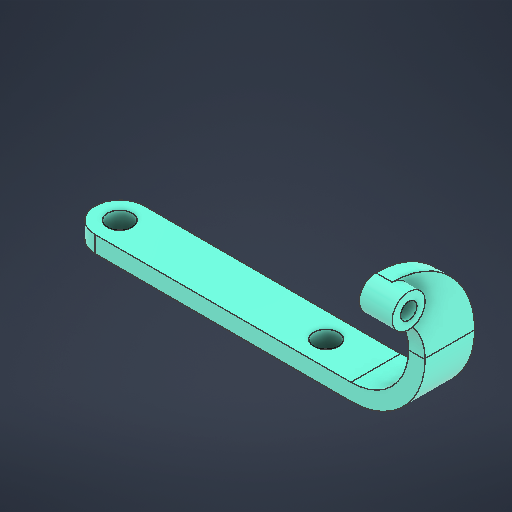
# Autodesk Inventor part: electronics_holder2
Saved by Autodesk Inventor 2026.1 (Build 301233000, 233)
## iProperties
Created: 2025-12-23
Part Number: electronics_holder2
Material: Generic
Document SubType Name: Modeling
Designer: emanuel
Density: 1 g/cm^3
Appearance: Default
Author: emanuel
Autodesk Inventor part; units mm, degrees
ref_plane "YZ Plane" through (0, 0, 0) normal (1, 0, 0) x (0, 1, 0)
ref_plane "XZ Plane" through (0, 0, 0) normal (0, 1, 0) x (-1, 0, 0)
ref_plane "XY Plane" through (0, 0, 0) normal (0, 0, 1) x (1, 0, 0)
sketch "Sketch1" plane through (0, 0, 0) normal (0, 1, 0) x (-1, 0, 0)
  line L0 (0, 0) -> (-25, 0)
  circle A0 centre (0, 0) radius 1.5
  circle A1 centre (-25, 0) radius 1.5
  line L1 (0, 0) -> (3, 0)
  line L2 (3, 0) -> (3, 3)
  line L3 (3, 3) -> (0, 3)
  line L4 (0, 3) -> (0, 0)
  line L5 (-25, 0) -> (-40, 0)
  line L6 (-40, 0) -> (-40, -3)
  line L7 (-40, -3) -> (-25, -3)
  line L8 (-25, -3) -> (-25, 0)
  line L9 (3, 3) -> (-40, 3)
  line L10 (-40, 3) -> (-40, -3)
  line L11 (-40, -3) -> (3, -3)
  line L12 (3, -3) -> (3, 3)
  dimension "d0" = 25
  dimension "d1" = 3
  dimension "d2" = 3
  dimension "d3" = 3
  dimension "d4" = 3
  dimension "d5" = 15
  dimension "d6" = 3
  constraints: 26 end point, 6 parallel, 4 horizontal, 3 perpendicular, 2 centre point, 2 coincident
  measures "d0" distance of L0.start L0.end
  measures "d1" diameter of A0
  measures "d2" diameter of A1
  measures "d3" distance of L3.end L2.end
  measures "d4" distance of L2.end L1.end
  measures "d5" distance of L7.end L6.end
  measures "d6" distance of L6.end L5.end
extrude "Extrusion1" add sketch "Sketch1" along normal blind 2 contours A1 L5 L10 L9 L4 A0 L0 | L0 A0 L1 L12 L11 L8 A1 | A1 L8 L7 L6 L5 | L4 L3 L2 L1 A0
fillet "Fillet12" radius 3 2 edges at (-3, 1, 3) (-3, 1, -3)
sketch "Sketch5" plane through (0, 2, 0) normal (0, 1, 0) x (1, 0, 0)
  line L0 (40, -3) -> (40, 3) projected
  line L1 (40, 3) -> (0, 3) projected
  line L2 (40, -3) -> (38, -3)
  line L3 (38, -3) -> (38, 3)
  line L4 (38, 3) -> (40, 3)
  line L5 (40, 3) -> (40, -3)
  point P0 (0, 0)
  dimension "d34" = 2
  constraints: 8 end point, 2 parallel, 1 horizontal, 1 perpendicular, 1 point on line
  measures "d34" distance of L3.end L4.end
extrude "Extrusion5" add sketch "Sketch5" along normal blind 17
sketch "Sketch6" plane through (40, 0, 3) normal (1, 0, 0) x (0, 0, -1)
  line L0 (6, 0) -> (6, 19) projected
  line L1 (6, 19) -> (-4, 19)
  line L2 (-4, 19) -> (-4, 17)
  line L3 (-4, 17) -> (6, 17)
  line L4 (6, 17) -> (6, 19)
  line L5 (-4, 17) -> (-6, 17)
  line L6 (-6, 17) -> (-6, 15)
  line L7 (-6, 15) -> (-4, 15)
  line L8 (-4, 15) -> (-4, 17)
  line L9 (-6, 15) -> (6, 15)
  line L10 (6, 15) -> (6, 19)
  line L11 (6, 19) -> (-6, 19)
  line L12 (-6, 19) -> (-6, 15)
  circle A0 centre (-4, 17) radius 1
  point P0 (3, 0)
  point P1 (6, 15)
  dimension "d37" = 10
  dimension "d38" = 2
  dimension "d39" = 2
  dimension "d40" = 2
  dimension "d41" = 2
  constraints: 24 end point, 6 parallel, 3 horizontal, 3 perpendicular, 1 centre point, 1 coincident
  measures "d37" distance of L3.end L2.end
  measures "d38" distance of L2.end L1.end
  measures "d39" distance of L7.end L6.end
  measures "d40" distance of L6.end L5.end
  measures "d41" diameter of A0
extrude "Extrusion6" add sketch "Sketch6" against normal blind 2 contours L9 L8 A0 L3 L0 | L3 A0 L2 L1 L0 | L7 L6 L5 A0 L8 | L2 A0 L5 L12 L11
sketch "Sketch7" plane through (40, 0, 3) normal (1, 0, 0) x (0, 0, -1)
  line L0 (6, 19) -> (-6, 19) projected
  line L1 (0, 15) -> (-6, 15) projected
  line L2 (-6, 19) -> (-2, 19)
  line L3 (-2, 19) -> (-2, 15)
  line L4 (-2, 15) -> (-6, 15)
  line L5 (-6, 15) -> (-6, 19)
  circle A0 centre (-4, 17) radius 1
  point P0 (3, 0)
  dimension "d44" = 4
  constraints: 8 end point, 2 parallel, 1 centre point, 1 horizontal, 1 perpendicular, 1 point on line
  measures "d44" distance of L3.end L4.end
extrude "Extrusion7" add sketch "Sketch7" along normal blind 2
fillet "Fillet13" radius 2 4 edges at (41, 19, 5) (40, 19, 9) (41, 15, 5) (40, 15, 9)
fillet "Fillet14" radius 6.5 1 edges at (39, 15, 3)
fillet "Fillet15" radius 10 1 edges at (39, 19, -3)
fillet "Fillet16" radius 7 1 edges at (38, 2, 0)
fillet "Fillet17" radius 9 1 edges at (40, 0, 0)
body "Solid1"
